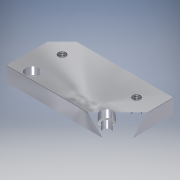
# Autodesk Inventor part: Portal-Column-v2-Top
Saved by Autodesk Inventor 2016 (Build 200138000, 138)
## iProperties
Created: 2015-10-26
Part Number: Portal-Column-v2-Top
Material: Aluminum 6061
Document SubType Name: Modeling
Designer: as
Mass: 37.1254 g
Surface Area: 54.1952 cm^2
Volume: 13.7501 cm^3
Density: 2.7 g/cm^3
Appearance: Aluminum - Flat
Author: as
Autodesk Inventor part; units mm, degrees
ref_plane "YZ Plane" through (0, 0, 0) normal (1, 0, 0) x (0, 1, 0)
ref_plane "XZ Plane" through (0, 0, 0) normal (0, 1, 0) x (-1, 0, 0)
ref_plane "XY Plane" through (0, 0, 0) normal (0, 0, 1) x (1, 0, 0)
sketch "Sketch1" plane through (0, 0, 0) normal (0, 0, 1) x (1, 0, 0)
  line L0 (0, 0) -> (60, 0)
  line L1 (60, 0) -> (60, 30)
  line L2 (60, 30) -> (0, 30)
  line L3 (0, 30) -> (0, 0)
  dimension "d0" = 60
  dimension "d1" = 30
  constraints: 8 end point, 2 parallel, 1 horizontal, 1 perpendicular
  measures "d0" distance of L2.end L1.end
  measures "d1" distance of L1.end L0.end
extrude "Extrusion1" add sketch "Sketch1" along normal blind 8
sketch "Sketch2" plane through (0, 0, 8) normal (0, 0, 1) x (1, 0, 0)
  circle A0 centre (10, 4) radius 2 projected
  circle A1 centre (50, 4) radius 2 projected
  point P0 (0, 0)
hole "Hole1" at (10, 4, 8) at (50, 4, 8) direction (0, 0, -1) diameter 4.5 end through all counterbore diameter 7 counterbore depth 4
sketch "Sketch3" plane through (0, 0, 8) normal (0, 0, 1) x (1, 0, 0)
  line L0 (0, 0) -> (60, 0) construction
  line L1 (30, 0) -> (30, 50) construction
  line L2 (30, 0) -> (80, 0) construction
  line L3 (-6.3387, 20) -> (66.0929, 20) construction
  line L4 (0, 30) -> (0, 0) projected
  line L5 (60, 0) -> (60, 30) projected
  point P0 (50, 20)
  point P1 (10, 20)
  dimension "d11" = 50
  dimension "d12" = 90
  dimension "d13" = 20
  dimension "d14" = 10
  dimension "d15" = 10
  constraints: 6 end point, 2 horizontal, 2 point on line, 1 midpoint, 1 perpendicular, 1 vertical
  measures "d11" distance of L1.start L1.end
  measures "d12" angle of L2 L1
  measures "d13" distance between parallel lines of L0 L3
  measures "d14" distance from line of L4 point (10, 20)
  measures "d15" distance from line of L5 point (50, 20)
hole "Hole2" at (50, 20, 8) at (10, 20, 8) direction (0, 0, -1) diameter 4.134 end through all thread size "M5x0.8" class "6H" standard "ISO Metric profile"
chamfer "Chamfer1" distance 0.1 angle 45 12 edges at (60, 15, 8) (30, 30, 8) (30, 0, 8) (0, 15, 8) (0, 15, 0) (30, 0, 0) (0, 0, 4) (60, 0, 4) (60, 15, 0) (60, 30, 4) (30, 30, 0) (0, 30, 4)
equation "\"d15\" = d14"
body "Solid1"
